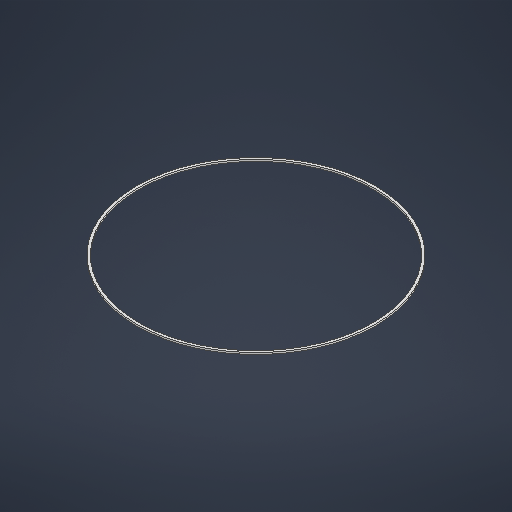
# Autodesk Inventor part: camera_base_test_print
Saved by Autodesk Inventor 2026.2 (Build 302298000, 298)
## iProperties
Created: 2026-02-25
Part Number: camera_base_test_print
Material: Generic
Document SubType Name: Modeling
Designer: Tathagata Sikdar
Density: 1 g/cm^3
Appearance: Default
Author: Tathagata Sikdar
Autodesk Inventor part; units mm, degrees
ref_plane "YZ Plane" through (0, 0, 0) normal (1, 0, 0) x (0, 1, 0)
ref_plane "XZ Plane" through (0, 0, 0) normal (0, 1, 0) x (-1, 0, 0)
ref_plane "XY Plane" through (0, 0, 0) normal (0, 0, 1) x (1, 0, 0)
sketch "Sketch1" plane through (0, 0, 0) normal (0, 1, 0) x (-1, 0, 0)
  line L0 (0, -60.0444) -> (52, 30.0222) construction
  line L1 (52, 30.0222) -> (-52, 30.0222) construction
  line L2 (-52, 30.0222) -> (0, -60.0444) construction
  line L3 (-26, -15.0111) -> (52, 30.0222) construction
  line L4 (0, -60.0444) -> (0, 30.0222) construction
  circle A0 centre (0, -60.0444) radius 2
  circle A1 centre (-52, 30.0222) radius 2
  circle A2 centre (52, 30.0222) radius 2
  circle A3 centre (0, 0) radius 68.5444
  line L5 (86.3467, 1.8023) -> (86.3467, 82.3467)
  line L6 (-86.3467, 1.8023) -> (-86.3467, 82.3467)
  line L7 (82.3467, 86.3467) -> (-82.3467, 86.3467)
  circle A4 centre (52, 30.0222) radius 5.75
  circle A5 centre (52, 30.0222) radius 3.75
  circle A6 centre (-52, 30.0222) radius 3.75
  circle A7 centre (-52, 30.0222) radius 5.75
  circle A8 centre (0, -60.0444) radius 3.75
  circle A9 centre (0, -60.0444) radius 5.75
  circle A10 centre (-82.3467, 82.3467) radius 2
  circle A11 centre (82.3467, 82.3467) radius 2
  circle A12 centre (0, -80.5444) radius 2
  arc A13 (-86.3467, 1.8023) -> (86.3467, 1.8023) centre (0, 1.8023) ccw
  line L8 (84.9267, 1.8023) -> (84.9267, 75.9404)
  arc A14 (78.934, 82.123) -> (82.123, 78.934) centre (82.3467, 82.3467) ccw
  line L9 (75.9404, 84.9267) -> (-75.9404, 84.9267)
  arc A15 (-82.123, 78.934) -> (-78.934, 82.123) centre (-82.3467, 82.3467) ccw
  line L10 (-84.9267, 75.9404) -> (-84.9267, 1.8023)
  arc A16 (3.4014, -80.1879) -> (-3.4014, -80.1879) centre (0, -80.5444) ccw
  arc A17 (-82.123, 78.934) -> (-84.9267, 75.9404) centre (-81.9267, 75.9404) ccw
  arc A18 (-75.9404, 84.9267) -> (-78.934, 82.123) centre (-75.9404, 81.9267) ccw
  arc A19 (78.934, 82.123) -> (75.9404, 84.9267) centre (75.9404, 81.9267) ccw
  arc A20 (84.9267, 75.9404) -> (82.123, 78.934) centre (81.9267, 75.9404) ccw
  arc A21 (6.6188, -82.8661) -> (84.9267, 1.8023) centre (0, 1.8023) ccw
  arc A22 (-84.9267, 1.8023) -> (-6.6188, -82.8661) centre (0, 1.8023) ccw
  line L11 (80.7667, 1.8023) -> (80.7667, 74.1638)
  arc A23 (75.1175, 80.0674) -> (80.0674, 75.1175) centre (82.3467, 82.3467) ccw
  line L12 (74.1638, 80.7667) -> (-74.1638, 80.7667)
  arc A24 (-80.0674, 75.1175) -> (-75.1175, 80.0674) centre (-82.3467, 82.3467) ccw
  line L13 (-80.7667, 74.1638) -> (-80.7667, 1.8023)
  arc A25 (-80.7667, 1.8023) -> (-8.1443, -78.5528) centre (0, 1.8023) ccw
  arc A26 (7.106, -77.9059) -> (-7.106, -77.9059) centre (0, -80.5444) ccw
  arc A27 (8.1443, -78.5528) -> (80.7667, 1.8023) centre (0, 1.8023) ccw
  arc A28 (-80.0674, 75.1175) -> (-80.7667, 74.1638) centre (-79.7667, 74.1638) ccw
  arc A29 (-74.1638, 80.7667) -> (-75.1175, 80.0674) centre (-74.1638, 79.7667) ccw
  arc A30 (75.1175, 80.0674) -> (74.1638, 80.7667) centre (74.1638, 79.7667) ccw
  arc A31 (80.7667, 74.1638) -> (80.0674, 75.1175) centre (79.7667, 74.1638) ccw
  arc A32 (7.106, -77.9059) -> (8.1443, -78.5528) centre (8.0434, -77.5579) ccw
  arc A33 (-8.1443, -78.5528) -> (-7.106, -77.9059) centre (-8.0434, -77.5579) ccw
  arc A34 (-6.6188, -82.8661) -> (-3.4014, -80.1879) centre (-6.385, -79.8752) ccw
  arc A35 (3.4014, -80.1879) -> (6.6188, -82.8661) centre (6.385, -79.8752) ccw
  arc A36 (86.3467, 82.3467) -> (82.3467, 86.3467) centre (82.3467, 82.3467) ccw
  arc A37 (-82.3467, 86.3467) -> (-86.3467, 82.3467) centre (-82.3467, 82.3467) ccw
  circle A38 centre (61.8467, 61.8467) radius 17.5 construction
  line L14 (-82.3467, 82.3467) -> (-86.3467, 86.3467) construction
  circle A39 centre (-84.468, 84.468) radius 1 construction
  circle A40 centre (61.8467, 61.8467) radius 18.92 construction
  line L15 (0, 0) -> (82.3467, 82.3467) construction
  circle A41 centre (0, 0) radius 69.9644
  arc A42 (73.8614, 79.3467) -> (79.3467, 73.8614) centre (82.3467, 82.3467) ccw
  line L16 (73.8614, 79.3467) -> (-73.8614, 79.3467)
  arc A43 (-79.3467, 73.8614) -> (-73.8614, 79.3467) centre (-82.3467, 82.3467) ccw
  line L17 (-79.3467, 73.8614) -> (-79.3467, 1.8023)
  arc A44 (-79.3467, 1.8023) -> (-8.3178, -77.1073) centre (0, 1.8023) ccw
  arc A45 (8.3178, -77.1073) -> (-8.3178, -77.1073) centre (0, -80.5444) ccw
  arc A46 (8.3178, -77.1073) -> (79.3467, 1.8023) centre (0, 1.8023) ccw
  line L18 (79.3467, 1.8023) -> (79.3467, 73.8614)
  point P0 (0, -84.5444)
  point P1 (84.9267, 84.5917)
  point P2 (80.1017, 84.9267)
  point P3 (-80.1017, 84.9267)
  point P4 (-84.9267, 80.1017)
  point P5 (0, -68.5444)
  dimension "d0" = 4
  dimension "d1" = 104
  dimension "d2" = 6.5
  dimension "d28" = 11.5
  dimension "d29" = 7.5
  dimension "d40" = 4
  dimension "d45" = 1.42
  dimension "d47" = 1.42
  dimension "d48" = 1.42
  dimension "d49" = 1.42
  dimension "d50" = 1.42
  dimension "d61" = 4.16
  dimension "d64" = 1
  dimension "d70" = 4
  dimension "d87" = 3
  dimension "d90" = 12
  dimension "ReservoirID" = 35
  dimension "d109" = 45
  dimension "d110" = 2
  dimension "d112" = 37.84
  dimension "d114" = 45
  constraints: 65 point on circle, 46 centre point, 38 end point, 36 tangent, 20 equal radius, 13 coincident, 8 point on line, 5 concentric, 4 horizontal alignment, 4 vertical alignment, 3 horizontal, 3 vertical, 2 equal length, 2 midpoint, 1 parallel, 19 other
  measures "d0" diameter of A0
  measures "d1" distance of L0.end L1.end
  measures "d28" diameter of A4
  measures "d29" diameter of A5
  measures "d40" distance of point (0, -84.544) A12.centre
  measures "d45" distance between parallel lines of L7 L9
  measures "d47" distance between parallel lines of L5 L8
  measures "d48" radial gap between concentric circles of A16 A12
  measures "d49" radial gap between concentric circles of A10 A15
  measures "d50" radial gap between concentric circles of A11 A14
  measures "d61" radial gap between concentric circles of A21 A27
  measures "d64" radius of A28
  measures "d70" radius of A36
  measures "d87" radius of A20
  measures "d90" distance of A12.centre point (0, -68.544)
  measures "ReservoirID" diameter of A38
  measures "d109" angle of L7 L14
  measures "d110" diameter of A39
  measures "d112" diameter of A40
  measures "d114" angle of L15 L4
extrude "Extrusion6" add sketch "Sketch1" along normal blind 1 contours A41
body "Solid4"
